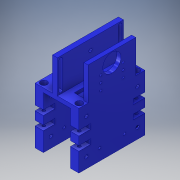
# Autodesk Inventor part: КВ33.044.501 - Каретка оси Y
Saved by Autodesk Inventor 2019 (Build 230136000, 136)
## iProperties
Created: 2019-07-21
Part Number: КВ33.044.501 - Каретка оси Y
Material: Пластик АБС
Document SubType Name: Modeling
Designer: Петров Иван
Density: 1.06 g/cm^3
Appearance: Синий — малярная краска — глянцевая
Author: Петров Иван
Autodesk Inventor part; units mm, degrees
ref_plane "YZ Plane" through (0, 0, 0) normal (1, 0, 0) x (0, 1, 0)
ref_plane "XZ Plane" through (0, 0, 0) normal (0, 1, 0) x (-1, 0, 0)
ref_plane "XY Plane" through (0, 0, 0) normal (0, 0, 1) x (1, 0, 0)
sketch "Эскиз1" plane through (0, 0, 0) normal (1, 0, 0) x (0, 1, 0)
  line L0 (-34, 40) -> (34, 40)
  line L1 (34, 40) -> (34, -40)
  line L2 (34, -40) -> (-34, -40)
  line L3 (-34, -40) -> (-34, 40)
  line L4 (-34, 40) -> (34, -40) construction
  line L5 (34, 40) -> (-34, -40) construction
  line L6 (0, 0) -> (0, 31)
  line L7 (0, 31) -> (21.3, 31)
  line L8 (0, 31) -> (-21.3, 31)
  line L9 (0, 0) -> (0, -31)
  line L10 (0, -31) -> (21.3, -31)
  line L11 (0, -31) -> (-21.3, -31)
  circle A0 centre (21.3, 31) radius 2.1
  circle A1 centre (-21.3, 31) radius 2.1
  circle A2 centre (21.3, -31) radius 2.1
  circle A3 centre (-21.3, -31) radius 2.1
  dimension "d0" = 68
  dimension "d1" = 80
  dimension "d2" = 21.3
  dimension "d3" = 21.3
  dimension "d4" = 31
  dimension "d5" = 31
  dimension "d6" = 21.3
  dimension "d7" = 21.3
  dimension "d8" = 4.2
  dimension "d9" = 4.2
  dimension "d10" = 4.2
  dimension "d11" = 4.2
  constraints: 24 end point, 4 centre point, 4 coincident, 3 horizontal, 3 perpendicular, 2 midpoint, 2 parallel, 2 vertical
  measures "d0" distance of L1.end L2.end
  measures "d1" distance of L0.end L1.end
  measures "d2" distance of L6.end L7.end
  measures "d3" distance of L6.end L8.end
  measures "d4" distance of L6.start L6.end
  measures "d5" distance of L6.start L9.end
  measures "d6" distance of L9.end L10.end
  measures "d7" distance of L9.end L11.end
  measures "d8" diameter of A0
  measures "d9" diameter of A1
  measures "d10" diameter of A2
  measures "d11" diameter of A3
extrude "Выдавливание1" add sketch "Эскиз1" along normal blind 10
sketch "Эскиз2" plane through (10, 0, 0) normal (1, 0, 0) x (0, 0, -1)
  line L0 (-40, 34) -> (-40, -34) projected
  line L1 (-40, 0) -> (-40, 5)
  line L2 (-40, 0) -> (-26, 0)
  line L3 (-26, 0) -> (-26, 11)
  line L4 (-40, 5) -> (-26, 5)
  line L5 (-26, 5) -> (-26, 11)
  line L6 (-26, 11) -> (-40, 11)
  line L7 (-40, 11) -> (-40, 5)
  line L8 (-40, 0) -> (-40, -5)
  line L9 (-26, 0) -> (-26, -11)
  line L10 (-40, -5) -> (-26, -5)
  line L11 (-26, -5) -> (-26, -11)
  line L12 (-26, -11) -> (-40, -11)
  line L13 (-40, -11) -> (-40, -5)
  line L14 (40, -34) -> (40, 34) projected
  line L15 (40, 0) -> (40, 5)
  line L16 (40, 0) -> (26, 0)
  line L17 (26, 0) -> (26, 11)
  line L18 (26, 11) -> (40, 11)
  line L19 (40, 11) -> (40, 5)
  line L20 (40, 5) -> (26, 5)
  line L21 (26, 5) -> (26, 11)
  line L22 (26, 0) -> (26, -11)
  line L23 (40, 0) -> (40, -5)
  line L24 (26, -11) -> (40, -11)
  line L25 (40, -11) -> (40, -5)
  line L26 (40, -5) -> (26, -5)
  line L27 (26, -5) -> (26, -11)
  point P0 (0, 0)
  dimension "d14" = 5
  dimension "d15" = 14
  dimension "d16" = 11
  dimension "d17" = 5
  dimension "d18" = 11
  dimension "d19" = 5
  dimension "d20" = 14
  dimension "d21" = 11
  dimension "d22" = 11
  dimension "d23" = 5
  constraints: 52 end point, 8 parallel, 7 perpendicular, 5 horizontal, 4 point on line, 2 midpoint, 2 vertical
  measures "d14" distance of L1.start L1.end
  measures "d15" distance of L1.start L2.end
  measures "d16" distance of L2.end L3.end
  measures "d17" distance of L1.start L8.end
  measures "d18" distance of L2.end L9.end
  measures "d19" distance of L15.start L15.end
  measures "d20" distance of L15.start L16.end
  measures "d21" distance of L16.end L17.end
  measures "d22" distance of L16.end L22.end
  measures "d23" distance of L15.start L23.end
extrude "Выдавливание2" cut sketch "Эскиз2" against normal blind 10 contours L6 L3 L4 L0 | L10 L9 L12 L0 | L24 L22 L26 L14 | L20 L17 L18 L14
sketch "Эскиз3" plane through (0, 34, 40) normal (0, 1, 0) x (1, 0, 0)
  line L0 (0, 0) -> (10, 0) projected
  line L1 (5, 0) -> (5, 11.1)
  line L2 (0, 11.1) -> (10, 11.1) projected
  circle A0 centre (5, 5.55) radius 1.8
  line L3 (0, 80) -> (10, 80) projected
  line L4 (5, 80) -> (5, 68.9)
  line L5 (0, 68.9) -> (10, 68.9) projected
  circle A1 centre (5, 74.45) radius 1.8
  point P0 (0, 40)
  dimension "d26" = 3.6
  dimension "d29" = 3.6
  constraints: 6 midpoint, 4 end point, 2 centre point
  measures "d26" diameter of A0
  measures "d29" diameter of A1
extrude "Выдавливание3" cut sketch "Эскиз3" against normal through all
sketch "Эскиз4" plane through (0, 34, 40) normal (0, 1, 0) x (1, 0, 0)
  circle A0 centre (5, 5.55) radius 1.8 projected
  circle A1 centre (5, 5.55) radius 4
  circle A2 centre (5, 74.45) radius 1.8 projected
  circle A3 centre (5, 74.45) radius 4
  point P0 (0, 40)
  dimension "d30" = 8
  dimension "d31" = 8
  constraints: 2 centre point, 2 coincident
  measures "d30" diameter of A1
  measures "d31" diameter of A3
extrude "Выдавливание4" cut sketch "Эскиз4" against normal blind 10
sketch "Эскиз5" plane through (10, 0, 0) normal (1, 0, 0) x (0, 0, -1)
  line L0 (0, 0) -> (0, 18)
  line L1 (0, 18) -> (0, 20)
  line L2 (0, 20) -> (-15, 20)
  line L3 (-15, 20) -> (15, 20)
  circle A0 centre (-15, 20) radius 1.5
  circle A1 centre (15, 20) radius 1.5
  line L4 (0, 0) -> (6.6954, 0)
  line L5 (0, -18) -> (0, -20)
  line L6 (0, -20) -> (-15, -20)
  line L7 (-15, -20) -> (15, -20)
  circle A2 centre (-15, -20) radius 1.5
  circle A3 centre (15, -20) radius 1.5
  dimension "d34" = 18
  dimension "d35" = 2
  dimension "d36" = 15
  dimension "d37" = 30
  dimension "d38" = 3
  dimension "d39" = 3
  constraints: 16 end point, 6 symmetric about line, 4 centre point, 4 coincident, 3 point on line, 2 horizontal, 1 vertical, 2 other
  measures "d34" distance of L0.start L0.end
  measures "d35" distance of L0.end L1.end
  measures "d36" distance of L1.end L2.end
  measures "d37" distance of L2.end L3.end
  measures "d38" diameter of A0
  measures "d39" diameter of A1
extrude "Выдавливание5" cut sketch "Эскиз5" against normal blind 10 contours A2 | A3
sketch "Эскиз6" plane through (10, 0, 0) normal (1, 0, 0) x (0, 0, -1)
  circle A0 centre (15, -20) radius 1.5 projected
  circle A1 centre (-15, -20) radius 1.5 projected
  circle A2 centre (-31, 21.3) radius 2.1 projected
  circle A3 centre (-31, -21.3) radius 2.1 projected
  circle A4 centre (31, 21.3) radius 2.1 projected
  circle A5 centre (31, -21.3) radius 2.1 projected
  line L0 (-40, 11) -> (-26, 11) projected
  line L1 (-26, 11) -> (-26, 5) projected
  line L2 (-26, 5) -> (-40, 5) projected
  line L3 (-40, 5) -> (-40, -5) projected
  line L4 (-40, -5) -> (-26, -5) projected
  line L5 (-26, -5) -> (-26, -11) projected
  line L6 (-26, -11) -> (-40, -11) projected
  line L7 (-40, -11) -> (-40, -34) projected
  line L8 (-40, -34) -> (40, -34) projected
  line L9 (40, -34) -> (40, -11) projected
  line L10 (40, -11) -> (26, -11) projected
  line L11 (26, -11) -> (26, -5) projected
  line L12 (26, -5) -> (40, -5) projected
  line L13 (40, -5) -> (40, 5) projected
  line L14 (40, 5) -> (26, 5) projected
  line L15 (26, 5) -> (26, 11) projected
  line L16 (26, 11) -> (40, 11) projected
  line L17 (40, 11) -> (40, 34) projected
  line L18 (40, 34) -> (-40, 34) projected
  line L19 (-40, 34) -> (-40, 11) projected
  point P0 (0, 0)
sketch "Эскиз8" plane through (0, 0, 0) normal (-1, 0, 0) x (0, 0, 1)
  line L0 (-40, 34) -> (-40, 11) projected
  line L1 (40, 11) -> (40, 34) projected
  line L2 (-40, 34) -> (40, 34)
  line L3 (40, 34) -> (40, 29)
  line L4 (40, 29) -> (-40, 29)
  line L5 (-40, 29) -> (-40, 34)
  point P0 (0, 0)
  dimension "d46" = 5
  constraints: 8 end point, 2 parallel, 1 horizontal, 1 perpendicular, 1 point on line
  measures "d46" distance of L2.end L3.end
extrude "Выдавливание7" add sketch "Эскиз8" along normal blind 33
sketch "Эскиз13" plane through (-33, 0, 0) normal (-1, 0, 0) x (0, 0, 1)
  circle A0 centre (15, -20) radius 1.5
  circle A1 centre (-15, -20) radius 1.5
  circle A2 centre (-31, 21.3) radius 2.1
  circle A3 centre (-31, -21.3) radius 2.1
  circle A4 centre (31, 21.3) radius 2.1
  circle A5 centre (31, -21.3) radius 2.1
  line L0 (-40, 11) -> (-26, 11)
  line L1 (-26, 11) -> (-26, 5)
  line L2 (-26, 5) -> (-40, 5)
  line L3 (-40, 5) -> (-40, -5)
  line L4 (-40, -5) -> (-26, -5)
  line L5 (-26, -5) -> (-26, -11)
  line L6 (-26, -11) -> (-40, -11)
  line L7 (-40, -11) -> (-40, -34)
  line L8 (-40, -34) -> (40, -34)
  line L9 (40, -34) -> (40, -11)
  line L10 (40, -11) -> (26, -11)
  line L11 (26, -11) -> (26, -5)
  line L12 (26, -5) -> (40, -5)
  line L13 (40, -5) -> (40, 5)
  line L14 (40, 5) -> (26, 5)
  line L15 (26, 5) -> (26, 11)
  line L16 (26, 11) -> (40, 11)
  line L17 (40, 11) -> (40, 34)
  line L18 (40, 34) -> (-40, 34)
  line L19 (-40, 34) -> (-40, 11)
  point P0 (0, 0)
  point P1 (0, 0)
  constraints: 40 end point, 6 centre point
extrude "Выдавливание11" add sketch "Эскиз13" along normal blind 10
sketch "Эскиз14" plane through (10, 34, 40) normal (0, 1, 0) x (1, 0, 0)
  line L0 (0, 80) -> (-53, 80) projected
  line L1 (-26.5, 80) -> (-26.5, 69.4857)
  circle A0 centre (-5, 5.55) radius 4 projected
  circle A1 centre (-5, 74.45) radius 4 projected
  line L2 (0, 0) -> (-53, 0) projected
  line L3 (0, 80) -> (0, 0) projected
  line L4 (0, 80) -> (-53, 80) projected
  line L5 (-53, 0) -> (-53, 80) projected
  circle A2 centre (-5, 5.55) radius 1.8 projected
  circle A3 centre (-5, 74.45) radius 1.8 projected
  circle A4 centre (-48, 5.55) radius 1.8
  circle A5 centre (-48, 74.45) radius 1.8
  point P0 (-10, 40)
  constraints: 2 centre point, 2 end point, 2 symmetric about line, 1 midpoint, 1 vertical, 2 other
extrude "Выдавливание12" cut sketch "Эскиз14" against normal through all contours A4 | A5
sketch "Эскиз15" plane through (10, 34, 40) normal (0, 1, 0) x (1, 0, 0)
  circle A0 centre (-48, 74.45) radius 1.8 projected
  circle A1 centre (-48, 74.45) radius 4
  circle A2 centre (-48, 5.55) radius 1.8 projected
  circle A3 centre (-48, 5.55) radius 4
  point P0 (-10, 40)
  dimension "d65" = 8
  dimension "d66" = 8
  constraints: 2 centre point, 2 coincident
  measures "d65" diameter of A1
  measures "d66" diameter of A3
extrude "Выдавливание13" cut sketch "Эскиз15" against normal blind 20
sketch "Эскиз16" plane through (10, 34, 40) normal (0, 1, 0) x (1, 0, 0)
  circle A0 centre (-48, 74.45) radius 4 projected
  circle A1 centre (-48, 5.55) radius 4 projected
  circle A2 centre (-5, 5.55) radius 4 projected
  circle A3 centre (-5, 74.45) radius 4 projected
  line L0 (0, 0) -> (-53, 0) projected
  line L1 (0, 80) -> (0, 0) projected
  line L2 (0, 80) -> (-53, 80) projected
  line L3 (-53, 0) -> (-53, 80) projected
  point P0 (-10, 40)
sketch "Эскиз17" plane through (-33, -34, -40) normal (0, -1, 0) x (1, 0, 0)
  circle A0 centre (-5, 5.55) radius 4
  circle A1 centre (-5, 74.45) radius 4
  circle A2 centre (-5, 5.55) radius 1.8 projected
  line L0 (-5, 5.55) -> (-5, 18.1127)
  circle A3 centre (38, 74.45) radius 4
  circle A4 centre (38, 5.55) radius 4
  circle A5 centre (-5, 5.55) radius 4
  circle A6 centre (-5, 74.45) radius 4
  line L1 (-10, 0) -> (43, 0)
  line L2 (-10, 80) -> (-10, 0)
  line L3 (-10, 80) -> (43, 80)
  line L4 (43, 0) -> (43, 80)
  circle A7 centre (-5, 5.55) radius 1.8
  point P0 (33, 40)
  point P1 (-10, 40)
  point P2 (0, 40)
  constraints: 10 end point, 7 centre point, 1 symmetric about line, 1 vertical, 3 other
extrude "Выдавливание14" cut sketch "Эскиз17" against normal blind 20 contours A0 | A1 | A3 | A4
sketch "Эскиз25" plane through (10, 34, 40) normal (0, 1, 0) x (1, 0, 0)
  line L0 (-10, 68.9) -> (0, 68.9) projected
  line L1 (-10, 11.1) -> (0, 11.1) projected
  line L2 (-5, 68.9) -> (0, 68.9)
  line L3 (0, 68.9) -> (0, 11.1)
  line L4 (0, 11.1) -> (-5, 11.1)
  line L5 (-5, 11.1) -> (-5, 68.9)
  point P0 (-10, 40)
  constraints: 8 end point, 2 parallel, 1 horizontal, 1 midpoint, 1 perpendicular, 1 point on line
extrude "Выдавливание21" add sketch "Эскиз25" along normal blind 40
sketch "Эскиз26" plane through (10, 0, 0) normal (1, 0, 0) x (0, 0, -1)
  line L0 (-12.6, 44.2) -> (-14.9, 44.2)
  line L1 (-12.6, 44.2) -> (-12.6, 42.8)
  line L2 (-14.9, 42.8) -> (-12.6, 42.8)
  line L3 (-14.9, 36.2) -> (-14.9, 42.8)
  line L4 (-12.6, 36.2) -> (-14.9, 36.2)
  circle A0 centre (0, 62) radius 9.15
  circle A1 centre (0, 62) radius 1.5
  circle A2 centre (8, 26) radius 1.3
  circle A3 centre (13.5, 39.5) radius 1.3
  circle A4 centre (13.5, 31.5) radius 1.3
  circle A5 centre (13.5, 47.5) radius 1.3
  circle A6 centre (13.5, 55.5) radius 1.3
  circle A7 centre (-8, 26) radius 1.3
  circle A8 centre (-13.5, 39.5) radius 1.3
  circle A9 centre (-13.5, 31.5) radius 1.3
  circle A10 centre (-13.5, 47.5) radius 1.3
  circle A11 centre (-13.5, 55.5) radius 1.3
  line L5 (-0.1, 73.0198) -> (-0.1, 72.4796)
  line L6 (-7, 73.0198) -> (-0.1, 73.0198)
  arc A12 (-7, 73.0198) -> (-7.75, 72.9686) centre (-7, 67.5) ccw
  line L7 (-7.75, 70.5) -> (-7.75, 72.9686)
  arc A13 (-9.5, 68.75) -> (-7.75, 70.5) centre (-9.5, 70.5) ccw
  line L8 (-10, 68.75) -> (-9.5, 68.75)
  line L9 (-10, 31.1937) -> (-10, 68.75)
  arc A14 (-10, 31.1937) -> (-9.6078, 30.5055) centre (-9.2, 31.1937) ccw
  arc A15 (-9.6078, 30.5055) -> (-8.9945, 29.8922) centre (-10.5, 29) ccw
  arc A16 (-8.9945, 29.8922) -> (-8.3063, 29.5) centre (-8.3063, 30.3) ccw
  line L10 (8.3063, 29.5) -> (-8.3063, 29.5)
  arc A17 (8.3063, 29.5) -> (8.9945, 29.8922) centre (8.3063, 30.3) ccw
  arc A18 (9.6078, 30.5055) -> (8.9945, 29.8922) centre (10.5, 29) ccw
  arc A19 (8.9945, 29.8922) -> (9.6078, 30.5055) centre (10.5, 29) ccw
  line L11 (-11.3229, 68.75) -> (-10, 68.75)
  arc A20 (-11.3229, 68.75) -> (-11.5, 67.4989) centre (-6.9922, 67.4989) ccw
  line L12 (-11.5, 67.4989) -> (-11.5, 60)
  line L13 (-12.6, 60) -> (-11.5, 60)
  line L14 (-12.6, 58.8) -> (-12.6, 60)
  line L15 (-14.9, 58.8) -> (-12.6, 58.8)
  line L16 (-14.9, 52.2) -> (-14.9, 58.8)
  line L17 (-12.6, 52.2) -> (-14.9, 52.2)
  line L18 (-12.6, 50.8) -> (-12.6, 52.2)
  line L19 (-14.9, 50.8) -> (-12.6, 50.8)
  line L20 (-14.9, 44.2) -> (-14.9, 50.8)
  line L21 (-12.6, 44.2) -> (-14.9, 44.2)
  line L22 (-12.6, 42.8) -> (-12.6, 44.2)
  line L23 (-14.9, 42.8) -> (-12.6, 42.8)
  line L24 (-14.9, 36.2) -> (-14.9, 42.8)
  line L25 (-12.6, 36.2) -> (-14.9, 36.2)
  line L26 (-12.6, 34.8) -> (-12.6, 36.2)
  line L27 (-14.9, 34.8) -> (-12.6, 34.8)
  line L28 (-14.9, 28.2) -> (-14.9, 34.8)
  line L29 (-12.6, 28.2) -> (-14.9, 28.2)
  line L30 (-12.6, 26.9802) -> (-12.6, 28.2)
  arc A21 (-12.6, 26.9802) -> (-12.5198, 26.9) centre (-11.5, 28) ccw
  line L31 (-11.3, 26.9) -> (-12.5198, 26.9)
  line L32 (-11.3, 24.6) -> (-11.3, 26.9)
  line L33 (-4.7, 24.6) -> (-11.3, 24.6)
  line L34 (-4.7, 26.9) -> (-4.7, 24.6)
  line L35 (4.7, 26.9) -> (-4.7, 26.9)
  line L36 (4.7, 24.6) -> (4.7, 26.9)
  line L37 (11.3, 24.6) -> (4.7, 24.6)
  line L38 (11.3, 26.9) -> (11.3, 24.6)
  line L39 (12.5198, 26.9) -> (11.3, 26.9)
  arc A22 (12.5198, 26.9) -> (12.6, 26.9802) centre (11.5, 28) ccw
  line L40 (12.6, 28.2) -> (12.6, 26.9802)
  line L41 (14.9, 28.2) -> (12.6, 28.2)
  line L42 (14.9, 34.8) -> (14.9, 28.2)
  line L43 (12.6, 34.8) -> (14.9, 34.8)
  line L44 (12.6, 36.2) -> (12.6, 34.8)
  line L45 (14.9, 36.2) -> (12.6, 36.2)
  line L46 (14.9, 42.8) -> (14.9, 36.2)
  line L47 (12.6, 42.8) -> (14.9, 42.8)
  line L48 (12.6, 44.2) -> (12.6, 42.8)
  line L49 (14.9, 44.2) -> (12.6, 44.2)
  line L50 (14.9, 50.8) -> (14.9, 44.2)
  line L51 (12.6, 50.8) -> (14.9, 50.8)
  line L52 (12.6, 52.2) -> (12.6, 50.8)
  line L53 (14.9, 52.2) -> (12.6, 52.2)
  line L54 (14.9, 58.8) -> (14.9, 52.2)
  line L55 (12.6, 58.8) -> (14.9, 58.8)
  line L56 (12.6, 60) -> (12.6, 58.8)
  line L57 (11.5, 60) -> (12.6, 60)
  line L58 (11.5, 67.5) -> (11.5, 60)
  arc A23 (11.5, 67.5) -> (11.3229, 68.75) centre (6.9922, 67.4989) ccw
  line L59 (10, 68.75) -> (11.3229, 68.75)
  line L60 (9.5, 68.75) -> (10, 68.75)
  arc A24 (7.75, 70.5) -> (9.5, 68.75) centre (9.5, 70.5) ccw
  line L61 (7.75, 72.9686) -> (7.75, 70.5)
  arc A25 (7.75, 72.9686) -> (7, 73.0198) centre (7, 67.5) ccw
  line L62 (0.1, 73.0198) -> (7, 73.0198)
  line L63 (0.1, 72.4796) -> (0.1, 73.0198)
  arc A26 (-8.9945, 29.8922) -> (-9.6078, 30.5055) centre (-10.5, 29) ccw
  arc A27 (9.6078, 30.5055) -> (10, 31.1895) centre (9.2, 31.1937) ccw
  line L64 (10, 68.75) -> (10, 31.1895)
  line L65 (0, 0) -> (0, 74)
  line L66 (28.9, 74) -> (-28.9, 74) projected
  line L67 (0, 74) -> (0, 62)
  point P0 (0, 62)
  dimension "d102" = 12
  constraints: 134 end point, 32 point on circle, 28 centre point, 1 midpoint, 1 point on line
  measures "d102" distance of L65.end L67.end
extrude "Выдавливание22" cut sketch "Эскиз26" against normal blind 40 contours A0 L65 A1 | L65 A1 A0 | L65 A1 | A1 L65 | A3 | A5 | A6 | A8 | A10 | A11
sketch "Эскиз27" plane through (5, 34, -28.9) normal (-1, 0, 0) x (0, 0, 1)
  line L0 (57.8, 40) -> (0, 40) projected
  line L1 (0, 40) -> (5, 40)
  line L2 (5, 40) -> (5, 30)
  line L3 (5, 30) -> (0, 30)
  line L4 (0, 30) -> (0, 40)
  line L5 (57.8, 40) -> (52.8, 40)
  line L6 (52.8, 40) -> (52.8, 30)
  line L7 (52.8, 30) -> (57.8, 30)
  line L8 (57.8, 30) -> (57.8, 40)
  point P0 (28.9, -34)
  dimension "d105" = 5
  dimension "d106" = 10
  dimension "d107" = 5
  dimension "d108" = 10
  constraints: 16 end point, 4 parallel, 2 horizontal, 2 perpendicular
  measures "d105" distance of L2.end L3.end
  measures "d106" distance of L1.end L2.end
  measures "d107" distance of L7.end L6.end
  measures "d108" distance of L6.end L5.end
sketch "Эскиз28" plane through (-43, 34, -40) normal (0, 1, 0) x (1, 0, 0)
  line L0 (10, -11.1) -> (0, -11.1) projected
  line L1 (0, -11.1) -> (10, -11.1)
  line L2 (10, -11.1) -> (10, -16.1)
  line L3 (10, -16.1) -> (0, -16.1)
  line L4 (0, -16.1) -> (0, -11.1)
  line L5 (10, -68.9) -> (0, -68.9) projected
  line L6 (0, -68.9) -> (10, -68.9)
  line L7 (10, -68.9) -> (10, -63.9)
  line L8 (10, -63.9) -> (0, -63.9)
  line L9 (0, -63.9) -> (0, -68.9)
  point P0 (43, -40)
  dimension "d109" = 10
  dimension "d110" = 5
  dimension "d111" = 10
  dimension "d112" = 5
  constraints: 16 end point, 4 parallel, 3 point on line, 2 horizontal, 2 perpendicular
  measures "d109" distance of L2.end L3.end
  measures "d110" distance of L1.end L2.end
  measures "d111" distance of L8.end L7.end
  measures "d112" distance of L7.end L6.end
sketch "Эскиз29" plane through (-43, 34, -40) normal (0, 1, 0) x (1, 0, 0)
  line L0 (43, -11.1) -> (53, -11.1) projected
  line L1 (48, -11.1) -> (48, -68.9) projected
  line L2 (48, -11.1) -> (48, -68.9)
  circle A0 centre (40.9968, -58.9777) radius 1.5
  line L3 (33.923, -34.3302) -> (33.923, -66.4777)
  line L4 (33.923, -66.4777) -> (47.9968, -66.4777)
  line L5 (47.9968, -66.4777) -> (47.9968, -34.3302)
  line L6 (47.9968, -34.3302) -> (33.923, -34.3302)
  point P0 (43, -40)
  point P1 (40.9968, -50.4777)
  constraints: 10 end point, 1 centre point, 1 collinear, 1 midpoint
extrude "Выдавливание23" cut sketch "Эскиз29" against normal blind 4 contours A0 | L6 L5 L4 L3
sketch "Эскиз30" plane through (-43, 34, -40) normal (0, 1, 0) x (1, 0, 0)
  line L0 (43, -11.1) -> (53, -11.1) projected
  line L1 (48, -11.1) -> (28.26, -11.1)
  line L2 (43, 0) -> (10, 0) projected
  line L3 (53, -80) -> (0, -80) projected
  line L4 (27, 0) -> (21, 0)
  line L5 (21, 0) -> (21, -80)
  line L6 (21, -80) -> (27, -80)
  line L7 (27, -80) -> (27, 0)
  line L8 (48, -11.1) -> (48, -68.9) projected
  point P0 (43, -40)
  dimension "d115" = 19.74
  dimension "d116" = 6
  dimension "d119" = 21
  constraints: 10 end point, 2 parallel, 2 point on line, 1 collinear, 1 horizontal, 1 midpoint, 1 perpendicular
  measures "d115" distance of L1.start L1.end
  measures "d116" distance of L6.end L5.end
  measures "d119" distance between parallel lines of L8 L7
extrude "Выдавливание24" add sketch "Эскиз30" along normal blind 40
sketch "Эскиз31" plane through (-22, 34, -40) normal (-1, 0, 0) x (0, 0, 1)
  circle A0 centre (40, 28) radius 9.15 projected
  circle A1 centre (40, 28) radius 2
  point P0 (40, -34)
  dimension "d120" = 4
  constraints: 1 centre point, 1 coincident
  measures "d120" diameter of A1
extrude "Выдавливание25" cut sketch "Эскиз31" against normal blind 40 contours A1
sketch "Эскиз32" plane through (-16, 34, 40) normal (1, 0, 0) x (0, 0, -1)
  line L0 (0, 0) -> (0, 40) projected
  line L1 (0, 20) -> (4, 20)
  line L2 (4, 3.4608) -> (4, 36.5392) construction
  line L3 (6.1, 3.4608) -> (6.1, 36.5392)
  line L4 (1.9, 36.5392) -> (1.9, 3.4608)
  arc A0 (1.9, 3.4608) -> (6.1, 3.4608) centre (4, 3.4608) ccw
  arc A1 (6.1, 36.5392) -> (1.9, 36.5392) centre (4, 36.5392) ccw
  line L5 (80, 40) -> (0, 40) projected
  line L6 (40, 40) -> (40, 35.6564)
  line L7 (80, 20) -> (76, 20)
  line L8 (76, 3.4608) -> (76, 36.5392) construction
  line L9 (73.9, 3.4608) -> (73.9, 36.5392)
  line L10 (78.1, 36.5392) -> (78.1, 3.4608)
  arc A2 (73.9, 3.4608) -> (78.1, 3.4608) centre (76, 3.4608) ccw
  arc A3 (78.1, 36.5392) -> (73.9, 36.5392) centre (76, 36.5392) ccw
  point P0 (40, -34)
  dimension "d123" = 4
  dimension "d124" = 4.2
  constraints: 22 end point, 8 point on circle, 8 symmetric about line, 4 centre point, 4 tangent, 3 midpoint, 1 horizontal, 1 parallel, 1 perpendicular, 1 vertical, 2 other
  measures "d123" distance of L1.start L1.end
  measures "d124" diameter of A1
extrude "Выдавливание26" cut sketch "Эскиз32" against normal blind 40
sketch "Эскиз33" plane through (10, 0, 0) normal (1, 0, 0) x (0, 0, -1)
  circle A0 centre (0, 62) radius 2 projected
  circle A1 centre (0, 62) radius 11
  point P0 (0, 0)
  dimension "d127" = 22
  constraints: 1 centre point, 1 coincident
  measures "d127" diameter of A1
extrude "Выдавливание27" cut sketch "Эскиз33" against normal blind 6
equation "\"d3\" = d2"
equation "\"d5\" = d4"
equation "\"d6\" = d2"
equation "\"d7\" = d2"
equation "\"d9\" = d8"
equation "\"d10\" = d8"
equation "\"d11\" = d8"
equation "\"d17\" = d14"
equation "\"d18\" = d16"
equation "\"d19\" = d14"
equation "\"d21\" = d16"
equation "\"d22\" = d16"
equation "\"d23\" = d14"
